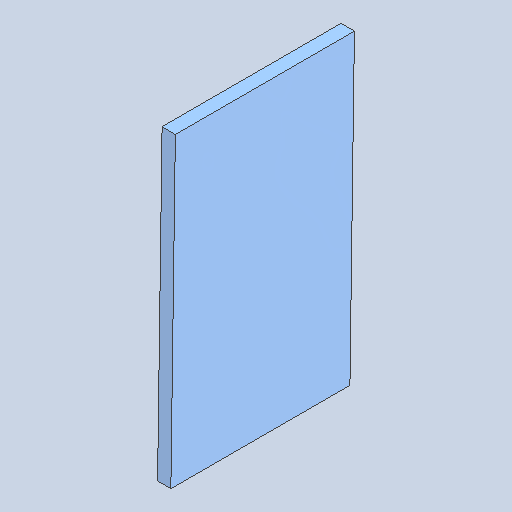
# Autodesk Inventor part: Ventana
Saved by Autodesk Inventor 2024 (Build 280153000, 153)
## iProperties
Created: 2024-04-05
Part Number: Ventana
Material: Genérico
Document SubType Name: Modeling
Designer: sergi
Density: 1 g/cm^3
Appearance: Valor por defecto
Author: sergi
Autodesk Inventor part; units mm, degrees
ref_plane "YZ Plane" through (0, 0, 0) normal (1, 0, 0) x (0, 1, 0)
ref_plane "XZ Plane" through (0, 0, 0) normal (0, 1, 0) x (-1, 0, 0)
sketch "Boceto1" plane through (0, 0, 0) normal (0, 0, 1) x (1, 0, 0)
  line L0 (133.9014, 2328.2978) -> (99.9894, -1.4554) projected
  line L1 (33.912, 2329.7532) -> (133.9014, 2328.2978) projected
  line L2 (0, 0) -> (33.912, 2329.7532) projected
  line L3 (0, 0) -> (99.9894, -1.4554) projected
ref_plane "Plano de trabajo1" through (0, -1.4554, 1350) normal (0, 0, -1) x (0, 1, 0)
extrude "Extrusión1" add sketch "Boceto1" along normal up to surface (1350 mm away)
